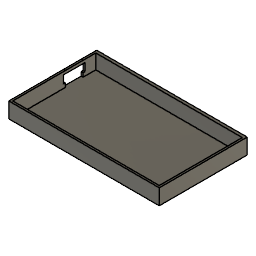
base (Autodesk Fusion 360 design; units mm, degrees)
part number: 2026-08-16-13-39-00-159
Autodesk Fusion 360 part; units mm, degrees
sketch "Sketch1" plane through (0, 0, 0) normal (0, 0, 1) x (1, 0, 0)
  line L0 (0, 0) -> (75, 0)
  line L1 (75, 0) -> (75, 42.5)
  line L2 (75, 42.5) -> (0, 42.5)
  line L3 (0, 0) -> (0, 27)
  line L4 (0, 42.5) -> (0, 36)
  line L5 (0, 27) -> (6, 27)
  line L6 (6, 27) -> (6, 36)
  line L7 (6, 36) -> (0, 36)
  line L8 (-1, 36) -> (-1, 44)
  line L9 (-1, 44) -> (76, 44)
  line L10 (76, 44) -> (76, -1)
  line L11 (76, -1) -> (-1, -1)
  line L12 (-1, -1) -> (-1, 27)
  line L13 (-1, 27) -> (-1, 36)
  line L14 (0, 36) -> (-1.5, 36)
  line L15 (-1.5, 36) -> (-1.5, 27)
  line L16 (-1.5, 27) -> (0, 27)
  dimension "d1" = 75
  dimension "d2" = 42.5
  dimension "d3" = 75
  dimension "d4" = 27
  dimension "d5" = 6.5
  constraint coincident L0.start L3.start
  constraint horizontal L0
  constraint perpendicular L0 L1
  constraint perpendicular L1 L2
  constraint perpendicular L0 L3
  constraint perpendicular L2 L4
  constraint perpendicular L3 L5
  constraint perpendicular L5 L6
  constraint perpendicular L7 L8
  constraint perpendicular L8 L9
  constraint perpendicular L9 L10
  constraint perpendicular L10 L11
  constraint perpendicular L5 L12
  constraint perpendicular L5 L13
  constraint perpendicular L8 L14
  constraint perpendicular L14 L15
  measures "d1" distance of L0.start L0.end
  measures "d2" distance of L0.end L1.end
  measures "d3" distance of L1.end L2.end
  measures "d4" distance of L0.start L3.end
  measures "d5" distance of L2.end L4.end
extrude "Extrude1" add sketch "Sketch1" along normal blind 8 contours L0 L1 L2 L3 L4 L8 L9 L10 L11 L12 L14 L16
sketch "Sketch2" plane through (-1, 0, 0) normal (-1, 0, 0) x (0, -1, 0)
  line L0 (-27, 0) -> (1, 0)
  line L1 (1, 0) -> (1, 8)
  line L2 (1, 8) -> (-27, 8)
  line L3 (-27, 8) -> (-27, 0)
  line L4 (-27, 0) -> (-27, 3)
  line L5 (-27, 3) -> (-36, 3)
  line L6 (-36, 3) -> (-36, 8)
  line L7 (-36, 8) -> (-27, 8)
  line L8 (-27, 3) -> (-27, 8)
  arc A0 (-36, 0.5) -> (-35.5, 0) centre (-35.5774, 0.4226) ccw
  arc A1 (-27.5, 0) -> (-27, 0.5) centre (-27.5, 0.5) ccw
  arc A2 (-35.5304, 3) -> (-36, 2.5) centre (-35.5852, 2.5809) ccw
  arc A3 (-27, 2.5) -> (-27.5, 3) centre (-27.431, 2.569) ccw
  line L9 (-35.5304, 3) -> (-36, 3)
  line L10 (-36, 2.5) -> (-36, 3)
  line L11 (-36, 0.5) -> (-36, 0)
  line L12 (-36, 0) -> (-35.5, 0)
  line L13 (-27.5, 0) -> (-27, 0)
  dimension "d8" = 3
  constraint coincident L0.start L3.end
  constraint perpendicular L0 L4
  constraint perpendicular L4 L5
  constraint perpendicular L5 L6
  constraint coincident L2.end L3.start
  constraint tangent L0 A1
  constraint coincident L4 A1.end
  constraint coincident L5 A2.start
  constraint coincident L3 A3.start
  constraint coincident L5 A3.end
  constraint perpendicular L9 L11
  constraint horizontal L12
  constraint tangent A1 L13
  measures "d8" distance of L0.start L4.end
extrude "Extrude2" add sketch "Sketch2" against normal blind 1 contours L3 L4 A1 L13 | L3 L4 L5 A3 | L5 A2 L9 L10 | A0 L11 L12
extrude "Extrude3" add sketch "Sketch2" against normal blind 1 contours L3 L5 L6 L7 L8 L9
sketch "Sketch3" plane through (0, 0, 0) normal (0, 0, 1) x (1, 0, 0)
  line L0 (0, 42.5) -> (75, 42.5)
  line L1 (75, 42.5) -> (75, 0)
  line L2 (75, 0) -> (0, 0)
  line L3 (0, 0) -> (0, 42.5)
  constraint horizontal L0
  constraint vertical L1
  constraint horizontal L2
  constraint vertical L3
extrude "Extrude4" add sketch "Sketch3" along normal blind 0.5
extrude "Extrude5" add 1 faces at (0, 30.1667, 0.3333) along direction (-1, 0, 0) blind 1
sketch "Sketch4" plane through (-1, 0, 0) normal (-1, 0, 0) x (0, -1, 0)
  line L0 (-37, 6.5) -> (-26, 6.5)
  line L1 (-26, 6.5) -> (-26, 2.5)
  line L2 (-26, 2.5) -> (-37, 2.5)
  line L3 (-37, 2.5) -> (-37, 6.5)
  constraint horizontal L0
  constraint vertical L1
  constraint horizontal L2
  constraint vertical L3
extrude "Extrude6" cut sketch "Sketch4" against normal blind 2
